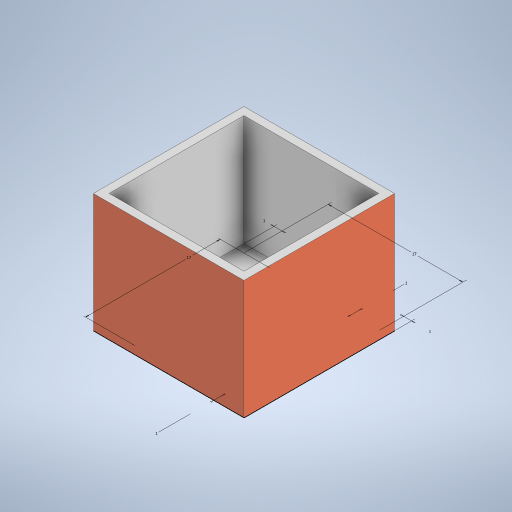
# Autodesk Inventor part: cubo
Saved by Autodesk Inventor 2023 (Build 270158000, 158)
## iProperties
Created: 2022-04-04
Part Number: cubo
Material: Genérico
Document SubType Name: Modeling
Designer: isaac
Density: 1 g/cm^3
Appearance: Valor por defecto
Author: isaac
Autodesk Inventor part; units mm, degrees
ref_plane "YZ Plane" through (0, 0, 0) normal (1, 0, 0) x (0, 1, 0)
ref_plane "XZ Plane" through (0, 0, 0) normal (0, 1, 0) x (-1, 0, 0)
ref_plane "XY Plane" through (0, 0, 0) normal (0, 0, 1) x (1, 0, 0)
sketch "Boceto1" plane through (0, 0, 0) normal (0, 1, 0) x (-1, 0, 0)
  line L0 (8.5, 8.5) -> (-8.5, 8.5)
  line L1 (-8.5, 8.5) -> (-8.5, -8.5)
  line L2 (-8.5, -8.5) -> (8.5, -8.5)
  line L3 (8.5, -8.5) -> (8.5, 8.5)
  line L4 (9.5, 9.5) -> (-9.5, 9.5)
  line L5 (-9.5, 9.5) -> (-9.5, -9.5)
  line L6 (-9.5, -9.5) -> (9.5, -9.5)
  line L7 (9.5, -9.5) -> (9.5, 9.5)
  point P0 (0, 0)
  point P1 (8.5, 0)
  point P2 (0, -8.5)
  dimension "d0" = 17
  dimension "d1" = 17
  dimension "d2" = 1
  dimension "d3" = 1
  dimension "d4" = 1
  dimension "d5" = 1
  constraints: 16 end point, 4 parallel, 2 horizontal, 2 midpoint, 2 perpendicular, 1 horizontal alignment, 1 vertical alignment
  measures "d0" distance between parallel lines of L2 L0
  measures "d1" distance between parallel lines of L1 L3
  measures "d2" distance between parallel lines of L3 L7
  measures "d3" distance between parallel lines of L4 L0
  measures "d4" distance between parallel lines of L5 L1
  measures "d5" distance between parallel lines of L6 L2
extrude "Extrusión1" add sketch "Boceto1" along normal blind 15
extrude "Extrusión2" add sketch "Boceto1" along normal blind 1 contours L3 L2 L1 L0
